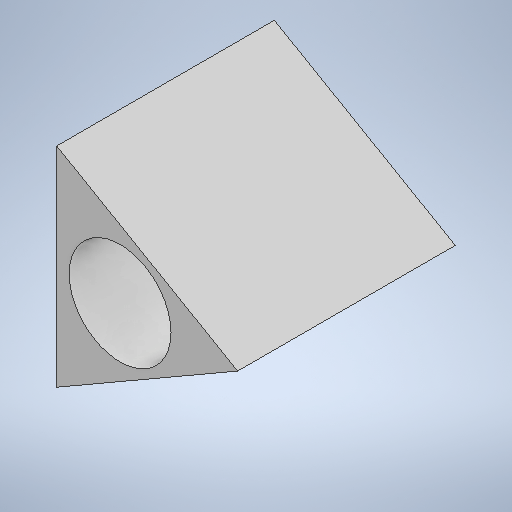
# Autodesk Inventor part: Triangle
Saved by Autodesk Inventor 2025.1 (Build 291241000, 241)
## iProperties
Created: 2025-04-04
Part Number: Triangle
Material: Generic
Document SubType Name: Modeling
Designer: victo
Density: 1 g/cm^3
Appearance: Default
Author: victo
Autodesk Inventor part; units mm, degrees
ref_plane "YZ Plane" through (0, 0, 0) normal (1, 0, 0) x (0, 1, 0)
ref_plane "XZ Plane" through (0, 0, 0) normal (0, 1, 0) x (-1, 0, 0)
ref_plane "XY Plane" through (0, 0, 0) normal (0, 0, 1) x (1, 0, 0)
sketch "Sketch1" plane through (0, 0, 0) normal (0, 0, 1) x (1, 0, 0)
  line L0 (0, 0) -> (-20.7846, 12)
  line L1 (-20.7846, 12) -> (-20.7846, -12)
  line L2 (-20.7846, -12) -> (0, 0)
  dimension "d7" = 24
  dimension "d8" = 24
  dimension "d9" = 24
  constraints: 6 end point, 1 vertical
  measures "d7" distance of L1.end L0.start
  measures "d8" distance of L0.start L0.end
  measures "d9" distance of L0.end L1.end
extrude "Extrusion1" add sketch "Sketch1" along normal blind 25
sketch "Sketch2" plane through (0, 0, 25) normal (0, 0, 1) x (1, 0, 0)
  circle A0 centre (-13.5, 0) radius 5.85
  point P0 (0, 0)
  dimension "d10" = 11.7
  dimension "d11" = 13.5
  dimension "d12" = 0
  constraints: 1 centre point
  measures "d10" diameter of A0
  measures "d11" distance of point (0, 0) A0.centre
  measures "d12" vertical distance of A0.centre point (0, 0)
extrude "Extrusion2" cut sketch "Sketch2" against normal up to surface (25 mm away)
equation "\"d7\" = d8"
equation "\"d9\" = d8"
body "Solid1"
